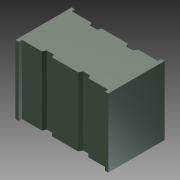
# Autodesk Inventor part: M20_ang1230TX-switch
Saved by Autodesk Inventor 2011 SP1 (Build 150282100, 282)
## iProperties
Created: 2013-12-24
Part Number: M20_ang1230TX-switch
Catalog Web Link: www.cadenas.de
Description: Angle Mount Miniature Rockers- Switch-Series M - Miniature Rockers
Vendor: NKKSWITCHES
Document SubType Name: Modeling
Designer: PARTuser1
Manufacturer: NKKSWITCHES
Density: 1 g/cm^3
Category: PARTsolutions
Company: NKKSWITCHES
Title: M20_ang1230TX-switch
Author: Cadenas PARTsolutions
Comments: Series M - Miniature Rockers
PSOL_IDENT_0: {$CADENAS_DATA\23d-libs\nkkswitches\toggle\m\parts\m_ang_t_switch.prj},233 {VTYP=3D},{NB=M20_ang1230
PSOL_IDENT_1: TX-switch},{LINA=M20_ang1230TX-switch},{NN=Angle Mount Miniature Rockers- Switch},{DATE=28.05.2007 0
PSOL_IDENT_2: 7:42:30},{GEOMDATE=28.05.2007 07:37:00},{VERSION=},{LINEID=10},{LINESUBID=-1},{WBVAR=PLS,CRCTS,FRM,T
PSOL_IDENT_3: RMNLS}  {NB=M20_ang1230TX-switch},{LINA=M20_ang1230TX-switch},{KT=DUMMY},{PN=M20_ang1230TX},{SRS=M20
PSOL_IDENT_4: },{PLS=1},{CRCTSALG='2','2 - ON/NONE/ON','3','3 - ON/OFF/ON','5','5 - ON/NONE/(ON)','8','8 - (ON)/OF
PSOL_IDENT_5: F/(ON)','9','9 - ON/OFF/(ON)','4', '4 - ON/ON/ON','6','6 - (ON)/ON/(ON)','7','7 - ON/ON/(ON)'},{CRCT
PSOL_IDENT_6: S=2},{FRMALG='TX', 'TX - Narrow Frame for Small Actuator', 'TZ'  , 'TZ - Wide Frame for Large Actuat
PSOL_IDENT_7: or'},{FRM=TX},{TRMNLSALG='30','30 - .150\" (3.81mm) Right Angle PC (1-3 Pole)','32','32 -  Right Ang
PSOL_IDENT_8: le PCB (1 Pole & 0.4VA Rating Only','40','40 - .150\" (3.81mm) Vertical PC (1-4 Pole)','45', '45 - .
PSOL_IDENT_9: 100\" (2.54mm) Vertical PC (1-4 Pole)'},{TRMNLS=30},{WIDTH=0.512},{HEIGHT=0.3877},{LENGTH=0.311},{A=
PSOL_IDENT_10: 0.15},{TRMNLNOH=1},{TRMNLOV=3},{LTRMNL=0.031},{POS=0},{POS2=0.185},{POS3=0},{D=0},{HOLES=0.185},{WH=
PSOL_IDENT_11: 0.00000},{D1=0.00000},{D2=0.00000}
CNS_NN: Angle Mount Miniature Rockers- Switch
CNS_NT: Series M - Miniature Rockers
CNS_NB: M20_ang1230TX-switch
CNS_NBSYN: $PN.-switch
CNS_LINA: M20_ang1230TX-switch
CNS_PN: M20_ang1230TX
CNS_SRS: M20
CNS_PLS: 1 - SPST/SPDT
CNS_CRCTSALG: '2','2 - ON/NONE/ON','3','3 - ON/OFF/ON','5','5 - ON/NONE/(ON)','8','8 - (ON)/OFF/(ON)','9','9 - ON/OFF/(ON)','4', '4 - ON/ON/ON','6','6 - (ON)/ON/(ON)','7','7 - ON/ON/(ON)'
CNS_CRCTS: 2 - ON/NONE/ON
CNS_FRMALG: 'TX', 'TX - Narrow Frame for Small Actuator', 'TZ'  , 'TZ - Wide Frame for Large Actuator'
CNS_FRM: TX - Narrow Frame for Small Actuator
CNS_TRMNLSALG: '30','30 - .150" (3.81mm) Right Angle PC (1-3 Pole)','32','32 -  Right Angle PCB (1 Pole & 0.4VA Rating Only','40','40 - .150" (3.81mm) Vertical PC (1-4 Pole)','45', '45 - .100" (2.54mm) Vertical PC (1-4 Pole)'
CNS_TRMNLS: 30 - .150" (3.81mm) Right Angle PC (1-3 Pole)
CNS_WIDTH: 0.512
CNS_HEIGHT: 0.388
CNS_LENGTH: 0.311
CNS_A: 0.150
CNS_TRMNLNOH: 1.000
CNS_TRMNLOV: 3.000
CNS_LTRMNL: 0.031
CNS_POS: 0.000
CNS_POS2: 0.185
CNS_POS3: 0.000
CNS_D: 0.000
CNS_HOLES: 0.185
CNS_WH: 0.00000
CNS_D1: 0.00000
CNS_D2: 0.00000
SUPPLIER: NKKSWITCHES
ARTICLENO: M20_ang1230TX-switch
BOMINFO: M20_ang1230TX-switch
CREATOR: CADENAS GmbH
Autodesk Inventor part; units mm, degrees
sketch "Sketch_2" plane through (0, -0.254, 0) normal (0, 1, 0) x (1, 0, 0)
  line L0 (-6.5024, -3.9497) -> (-6.0389, -3.9497)
  line L1 (-6.0389, -3.9497) -> (-6.0389, -3.4862)
  line L2 (-6.0389, -3.4862) -> (-3.2509, -3.4862)
  line L3 (-3.2509, -3.4862) -> (-3.0348, -3.0226)
  line L4 (-3.0348, -3.0226) -> (-2.0452, -3.0226)
  line L5 (-2.0452, -3.0226) -> (-1.8291, -3.4862)
  line L6 (-1.8291, -3.4862) -> (1.8291, -3.4862)
  line L7 (1.8291, -3.4862) -> (2.0452, -3.0226)
  line L8 (2.0452, -3.0226) -> (3.0348, -3.0226)
  line L9 (3.0348, -3.0226) -> (3.2509, -3.4862)
  line L10 (3.2509, -3.4862) -> (6.0389, -3.4862)
  line L11 (6.0389, -3.4862) -> (6.0389, -3.9497)
  line L12 (6.0389, -3.9497) -> (6.5024, -3.9497)
  line L13 (6.5024, -3.9497) -> (6.5024, 3.9497)
  line L14 (6.5024, 3.9497) -> (6.0389, 3.9497)
  line L15 (6.0389, 3.9497) -> (6.0389, 3.4862)
  line L16 (6.0389, 3.4862) -> (3.2509, 3.4862)
  line L17 (3.2509, 3.4862) -> (3.0348, 3.0226)
  line L18 (3.0348, 3.0226) -> (2.0452, 3.0226)
  line L19 (2.0452, 3.0226) -> (1.8291, 3.4862)
  line L20 (1.8291, 3.4862) -> (-1.8291, 3.4862)
  line L21 (-1.8291, 3.4862) -> (-2.0452, 3.0226)
  line L22 (-2.0452, 3.0226) -> (-3.0348, 3.0226)
  line L23 (-3.0348, 3.0226) -> (-3.2509, 3.4862)
  line L24 (-3.2509, 3.4862) -> (-6.0389, 3.4862)
  line L25 (-6.0389, 3.4862) -> (-6.0389, 3.9497)
  line L26 (-6.0389, 3.9497) -> (-6.5024, 3.9497)
  line L27 (-6.5024, 3.9497) -> (-6.5024, -3.9497)
  constraints: 56 end point
extrude "Extrusion1" add sketch "Sketch_2" against normal blind 9.8476
sketch "Sketch_8" plane through (0, -9.5936, 0) normal (0, 1, 0) x (1, 0, 0)
  line L0 (-5.08, -0.889) -> (-4.318, -0.889)
  line L1 (-4.318, -0.889) -> (-4.318, 0.889)
  line L2 (-4.318, 0.889) -> (-5.08, 0.889)
  line L3 (-5.08, 0.889) -> (-5.08, -0.889)
  constraints: 8 end point
extrude "Extrusion2" cut sketch "Sketch_8" against normal blind 25.4
sketch "Sketch_5" plane through (0, -9.5936, 0) normal (0, 1, 0) x (1, 0, 0)
  line L0 (-0.381, -0.889) -> (0.381, -0.889)
  line L1 (0.381, -0.889) -> (0.381, 0.889)
  line L2 (0.381, 0.889) -> (-0.381, 0.889)
  line L3 (-0.381, 0.889) -> (-0.381, -0.889)
  constraints: 8 end point
extrude "Extrusion3" cut sketch "Sketch_5" against normal blind 25.4
sketch "Sketch_9" plane through (0, -9.5936, 0) normal (0, 1, 0) x (1, 0, 0)
  line L0 (4.318, -0.889) -> (5.08, -0.889)
  line L1 (5.08, -0.889) -> (5.08, 0.889)
  line L2 (5.08, 0.889) -> (4.318, 0.889)
  line L3 (4.318, 0.889) -> (4.318, -0.889)
  constraints: 8 end point
extrude "Extrusion4" cut sketch "Sketch_9" against normal blind 25.4
sketch "Sketch_19" plane through (0, -0.254, 0) normal (0, 1, 0) x (1, 0, 0)
  line L0 (-6.5024, -3.9497) -> (-6.0389, -3.9497)
  line L1 (-6.0389, -3.9497) -> (-6.0389, -3.4862)
  line L2 (-6.0389, -3.4862) -> (-3.2509, -3.4862)
  line L3 (-3.2509, -3.4862) -> (-3.0348, -3.0226)
  line L4 (-3.0348, -3.0226) -> (-2.0452, -3.0226)
  line L5 (-2.0452, -3.0226) -> (-1.8291, -3.4862)
  line L6 (-1.8291, -3.4862) -> (1.8291, -3.4862)
  line L7 (1.8291, -3.4862) -> (2.0452, -3.0226)
  line L8 (2.0452, -3.0226) -> (3.0348, -3.0226)
  line L9 (3.0348, -3.0226) -> (3.2509, -3.4862)
  line L10 (3.2509, -3.4862) -> (6.0389, -3.4862)
  line L11 (6.0389, -3.4862) -> (6.0389, -3.9497)
  line L12 (6.0389, -3.9497) -> (6.5024, -3.9497)
  line L13 (6.5024, -3.9497) -> (6.5024, 3.9497)
  line L14 (6.5024, 3.9497) -> (6.0389, 3.9497)
  line L15 (6.0389, 3.9497) -> (6.0389, 3.4862)
  line L16 (6.0389, 3.4862) -> (3.2509, 3.4862)
  line L17 (3.2509, 3.4862) -> (3.0348, 3.0226)
  line L18 (3.0348, 3.0226) -> (2.0452, 3.0226)
  line L19 (2.0452, 3.0226) -> (1.8291, 3.4862)
  line L20 (1.8291, 3.4862) -> (-1.8291, 3.4862)
  line L21 (-1.8291, 3.4862) -> (-2.0452, 3.0226)
  line L22 (-2.0452, 3.0226) -> (-3.0348, 3.0226)
  line L23 (-3.0348, 3.0226) -> (-3.2509, 3.4862)
  line L24 (-3.2509, 3.4862) -> (-6.0389, 3.4862)
  line L25 (-6.0389, 3.4862) -> (-6.0389, 3.9497)
  line L26 (-6.0389, 3.9497) -> (-6.5024, 3.9497)
  line L27 (-6.5024, 3.9497) -> (-6.5024, -3.9497)
  constraints: 56 end point
extrude "Extrusion5" cut sketch "Sketch_19" against normal blind 0.254
ref_plane "rot_XY" through (0, 6.6675, 0) normal (0, 0, 1) x (1, 0, 0)
ref_plane "rot_YZ" through (0, 6.6675, 0) normal (1, 0, 0) x (0, 1, 0)
ref_plane "rot_ZX" through (0, 6.6675, 0) normal (0, 1, 0) x (0, 0, 1)
ref_plane "to_cover_XY" through (0, -0.254, 0) normal (0, 1, 0) x (1, 0, 0)
ref_plane "to_cover_YZ" through (0, -0.254, 0) normal (1, 0, 0) x (0, 0, -1)
ref_plane "to_cover_ZX" through (0, -0.254, 0) normal (0, 0, -1) x (0, 1, 0)
ref_plane "to_terminals_XY" through (0, -9.5936, 0) normal (0, -1, 0) x (1, 0, 0)
ref_plane "to_terminals_YZ" through (0, -9.5936, 0) normal (1, 0, 0) x (0, 0, 1)
ref_plane "to_terminals_ZX" through (0, -9.5936, 0) normal (0, 0, 1) x (0, -1, 0)
body "Solid1"
